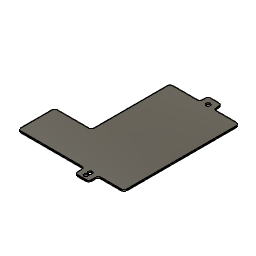
osborne 1 (Autodesk Fusion 360 design; units mm, degrees)
Autodesk Fusion 360 part; units mm, degrees
sketch "Sketch1" plane through (0, 0, 0) normal (0, 0, 1) x (1, 0, 0)
  circle A0 centre (45, 88.0004) radius 1.5
  circle A1 centre (45, 1.0004) radius 1.5
  circle A2 centre (45, -1.9996) radius 1.5
  line L0 (69, 85) -> (69, 4)
  line L1 (49.9968, 91.0004) -> (49.9968, 89)
  line L2 (51.9968, 87) -> (67, 87)
  line L3 (49.9966, -2.9996) -> (49.9966, 0)
  line L4 (51.9966, 2) -> (67, 2)
  line L5 (39.8987, 91.0004) -> (39.8987, 89)
  line L6 (37.8987, 87) -> (20, 87)
  line L7 (39.8987, -2.9996) -> (39.8987, 0.0092)
  line L8 (37.8987, 2.0092) -> (-7.1013, 2.0092)
  line L9 (-9.1013, 4.0092) -> (-9.1013, 27)
  line L10 (-7.1013, 29) -> (16, 29)
  line L11 (18, 31) -> (18, 85)
  line L12 (41.8987, 93.0004) -> (47.9968, 93.0004)
  line L13 (41.8987, -4.9996) -> (47.9966, -4.9996)
  arc A3 (41.8987, 93.0004) -> (39.8987, 91.0004) centre (41.8987, 91.0004) ccw
  arc A4 (49.9968, 91.0004) -> (47.9968, 93.0004) centre (47.9968, 91.0004) ccw
  arc A5 (37.8987, 87) -> (39.8987, 89) centre (37.8987, 89) ccw
  arc A6 (49.9968, 89) -> (51.9968, 87) centre (51.9968, 89) ccw
  arc A7 (39.8987, 0.0092) -> (37.8987, 2.0092) centre (37.8987, 0.0092) ccw
  arc A8 (39.8987, -2.9996) -> (41.8987, -4.9996) centre (41.8987, -2.9996) ccw
  arc A9 (47.9966, -4.9996) -> (49.9966, -2.9996) centre (47.9966, -2.9996) ccw
  arc A10 (51.9966, 2) -> (49.9966, 0) centre (51.9966, 0) ccw
  arc A11 (-7.1013, 29) -> (-9.1013, 27) centre (-7.1013, 27) ccw
  arc A12 (-9.1013, 4.0092) -> (-7.1013, 2.0092) centre (-7.1013, 4.0092) ccw
  arc A13 (16, 29) -> (18, 31) centre (16, 31) ccw
  arc A14 (20, 87) -> (18, 85) centre (20, 85) ccw
  arc A15 (69, 85) -> (67, 87) centre (67, 85) ccw
  arc A16 (67, 2) -> (69, 4) centre (67, 4) ccw
  dimension "d1" = 3
  dimension "d2" = 3
  dimension "d3" = 3
  dimension "d4" = 87
  dimension "d5" = 3
  dimension "d8" = 24
  dimension "d16" = 2
  dimension "d17" = 2
  dimension "d18" = 2
  dimension "d19" = 2
  dimension "d20" = 2
  dimension "d21" = 2
  dimension "d22" = 2
  dimension "d23" = 2
  dimension "d24" = 2
  dimension "d25" = 2
  dimension "d26" = 2
  dimension "d27" = 2
  dimension "d28" = 2
  dimension "d29" = 2
  constraint vertical L0
  constraint perpendicular L3 L13
  constraint tangent L5 A3
  constraint tangent L12 A3
  constraint tangent L1 A4
  constraint tangent L12 A4
  constraint tangent L5 A5
  constraint tangent L6 A5
  constraint tangent L1 A6
  constraint tangent L2 A6
  constraint tangent L8 A7
  constraint tangent L7 A7
  constraint tangent L7 A8
  constraint tangent L13 A8
  constraint tangent L3 A9
  constraint tangent L13 A9
  constraint tangent L3 A10
  constraint tangent L4 A10
  constraint tangent L9 A11
  constraint tangent L10 A11
  constraint tangent L8 A12
  constraint tangent L9 A12
  constraint tangent L10 A13
  constraint tangent L11 A13
  constraint tangent L6 A14
  constraint tangent L11 A14
  constraint tangent L2 A15
  constraint tangent L0 A15
  constraint tangent L4 A16
  constraint tangent L0 A16
  measures "d5" diameter of A0
  measures "d5" diameter of A1
  measures "d5" diameter of A2
  measures "d5" distance of A1.centre A2.centre
  measures "d8" distance of A0.centre L0
  measures "d16" radius of A3
  measures "d17" radius of A4
  measures "d18" radius of A5
  measures "d19" radius of A6
  measures "d20" radius of A7
  measures "d21" radius of A8
  measures "d22" radius of A9
  measures "d23" radius of A10
  measures "d24" radius of A11
  measures "d25" radius of A12
  measures "d26" radius of A13
  measures "d27" radius of A14
  measures "d28" radius of A15
  measures "d29" radius of A16
extrude "Extrude2" add sketch "Sketch1" along normal blind 1
